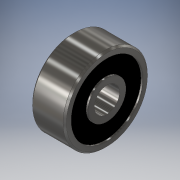
# Autodesk Inventor part: 623bearing
Saved by Autodesk Inventor 2017 (Build 210142000, 142)
## iProperties
Created: 2016-05-21
Part Number: 623bearing
Material: Glass
Document SubType Name: Modeling
Designer: brent
Density: 2.18 g/cm^3
Appearance: Steel - Polished
Author: brent
Autodesk Inventor part; units mm, degrees
ref_plane "YZ Plane" through (0, 0, 0) normal (1, 0, 0) x (0, 1, 0)
ref_plane "XZ Plane" through (0, 0, 0) normal (0, 1, 0) x (-1, 0, 0)
sketch "Sketch1" plane through (0, 0, 0) normal (0, 1, 0) x (-1, 0, 0)
  line L0 (0, 0) -> (4, 0)
  line L1 (4, 0) -> (4, -1.5)
  line L2 (4, -1.5) -> (0, -1.5)
  line L3 (0, -1.5) -> (0, 0)
  line L4 (4, -1.5) -> (0, -1.5)
  line L5 (0, -1.5) -> (0, -5)
  line L6 (0, -5) -> (4, -5)
  line L7 (4, -5) -> (4, -1.5)
  line L8 (4, -2.25) -> (3.8, -2.25)
  line L9 (3.8, -2.25) -> (3.8, -4.25)
  line L10 (3.8, -4.25) -> (4, -4.25)
  line L11 (4, -4.25) -> (4, -2.25)
  line L12 (0, -2.25) -> (0.2, -2.25)
  line L13 (0.2, -2.25) -> (0.2, -4.25)
  line L14 (0.2, -4.25) -> (0, -4.25)
  line L15 (0, -4.25) -> (0, -2.25)
  dimension "d0" = 4
  dimension "d1" = 1.5
  dimension "d2" = 4
  dimension "d3" = 3.5
  dimension "d4" = 0.75
  dimension "d5" = 0.75
  dimension "d6" = 0.2
  dimension "d7" = 0.2
  constraints: 32 end point, 8 parallel, 4 horizontal, 4 perpendicular, 4 point on line
  measures "d0" distance of L1.end L2.end
  measures "d1" distance of L0.end L1.end
  measures "d2" distance of L6.end L5.end
  measures "d3" distance of L5.end L4.end
  measures "d4" distance between parallel lines of L6 L14
  measures "d5" distance between parallel lines of L2 L12
  measures "d6" distance of L13.end L14.end
  measures "d7" distance of L9.end L10.end
revolve "Revolution1" add sketch "Sketch1" angle 360 about axis through (0, 0, 0) along (-1, 0, 0) contours L2 L7 L8 L9 L10 L6 L5 L14 L13 L12
ref_plane "Work Plane1" through (-2, 0, 0) normal (1, 0, 0) x (0, 0, -1)
sketch "Sketch2" plane through (-2, 0, 0) normal (1, 0, 0) x (0, 0, -1)
  circle A0 centre (0, 0) radius 4.25
  circle A1 centre (0, 0) radius 2.25
  circle A2 centre (-3.25, 0) radius 1
  line L0 (-3.25, 0) -> (0, 0) construction
  line L1 (-3.25, 0) -> (0, 0) construction
  dimension "d9" = 8.5
  dimension "d13" = 2
  constraints: 4 end point, 3 centre point, 3 coincident, 2 tangent, 1 collinear, 1 horizontal
  measures "d9" diameter of A0
  measures "d13" radial gap between concentric circles of A0 A1
extrude "Extrusion1" cut sketch "Sketch2" along normal mid plane 2.5 contours A2 | A0
extrude "Extrusion2" add sketch "Sketch2" along normal mid plane 2 separate body contours A2
fillet "Fillet1" radius 1 2 edges at (-1, 0, 4.25) (-3, 0, 4.25)
pattern_circular "Circular Pattern1" count 9 over 360 about axis through (-2, 0, 0) along (1, 0, 0) bodies 2
chamfer "Chamfer1" distance 0.2 angle 45 2 edges at (0, 0, 5) (-4, 0, 5)
equation "\"d7\" = d6"
body "Solid1"
body "Solid4"
